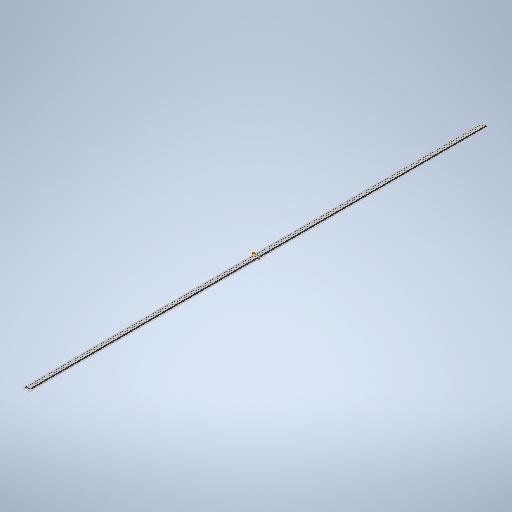
# Autodesk Inventor part: SP40-10 JUNTA INT CRISTAL 1023
Saved by Autodesk Inventor 2025 (Build 290162000, 162)
## iProperties
Created: 2026-01-18
Part Number: SP40-10 JUNTA INT CRISTAL 1023
Material: Caucho
Document SubType Name: Modeling
Designer: ROLANDO
Density: 0.93 g/cm^3
Appearance: Caucho - Negro
Author: ROLANDO
Autodesk Inventor part; units mm, degrees
ref_plane "YZ Plane" through (0, 0, 0) normal (1, 0, 0) x (0, 1, 0)
ref_plane "XZ Plane" through (0, 0, 0) normal (0, 1, 0) x (-1, 0, 0)
sketch "Boceto3" plane through (0, 0, 0) normal (0, 0, 1) x (1, 0, 0)
  line L0 (-15.1624, 32.0626) -> (-18.8843, 32.0626)
  line L1 (-13.7243, 33.4626) -> (-13.7243, 30.9626)
  line L2 (-13.7243, 30.9626) -> (-14.4343, 30.9626)
  line L3 (-14.4343, 30.9626) -> (-15.1624, 32.0626)
  arc A0 (-18.8843, 32.0626) -> (-21.6243, 29.3226) centre (-18.8843, 29.3226) ccw
  line L4 (-13.7243, 33.4626) -> (-10.2243, 33.4626)
  line L5 (-21.6243, 29.3226) -> (-21.6243, 26.5626)
  arc A1 (-10.2243, 33.4626) -> (-10.2243, 26.5626) centre (5.1794, 30.0126) ccw
  line L6 (-21.6243, 26.5626) -> (-21.1243, 26.5626)
  line L7 (-10.2243, 26.5626) -> (-10.7243, 26.5626)
  arc A2 (-10.7243, 26.5626) -> (-21.1243, 26.5626) centre (-15.9243, 23.1493) ccw
  dimension "d218" = 2.5
  dimension "d219" = 0.71
  dimension "d221" = 33.5
  dimension "d223" = 2.74
  dimension "d281" = 3.5
  dimension "d288" = 2.76
  dimension "d291" = 0.5
  dimension "d292" = 0.5
  constraints: 16 end point, 6 point on circle, 3 centre point, 3 horizontal, 2 vertical, 1 collinear, 1 perpendicular, 1 tangent
  measures "d218" distance of L1.start L1.end
  measures "d219" distance of L1.end L2.end
  measures "d221" angle of L1 L3
  measures "d223" radius of A0
  measures "d281" distance of L1.start L4.end
  measures "d288" distance of L5.start L5.end
  measures "d291" distance of L5.end L6.end
  measures "d292" distance of L7.start L7.end
extrude "Extrusión4" add sketch "Boceto3" against normal blind 1023.4
ref_plane "Plano de trabajo2" through (-10.2243, 33.4626, 0) normal (-1, 0, 0) x (0, 0, -1)
ref_plane "Plano de trabajo4" through (0, 0, -511.7) normal (0, 0, 1) x (1, 0, 0)
sketch "Boceto5" plane through (-10.2243, 33.4626, 0) normal (-1, 0, 0) x (0, 0, -1)
  line L0 (0, 0) -> (0, 6.9) projected
  line L1 (0, 6.9) -> (6.9, 0)
  line L2 (0, 0) -> (1023.4, 0) projected
  line L3 (6.9, 0) -> (0, 0)
  line L4 (0, 0) -> (0, 6.9)
  point P0 (0, 33.4626)
  dimension "d296" = 45
  constraints: 6 end point, 1 horizontal, 1 perpendicular, 1 point on line
  measures "d296" angle of L0 L1
extrude "Extrusión6" cut sketch "Boceto5" along normal through all
mirror "Simetría3" about plane through (0, 0, -511.7) normal (0, 0, 1) of "Extrusión6"
